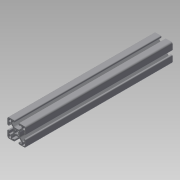
# Autodesk Inventor part: 1515-LS
Saved by Autodesk Inventor 2013 (Build 170138000, 138)
## iProperties
Created: 2014-04-23
Part Number: 1515-LS
Material: Generic
Document SubType Name: Modeling
Density: 1 g/cm^3
Vendor: 80/20 Inc.
Engineer: Ross Bowman
Designer: Ross Bowman
Catalog Web Link: 8020.net
Company: 80/20 Inc.
Author: Ross Bowman
Keywords: 80/20 , 8020 , T-Slot , Extrusion
Material: 6105-T5 Aluminum
Autodesk Inventor part; units mm, degrees
ref_plane "YZ Plane" through (0, 0, 0) normal (1, 0, 0) x (0, 1, 0)
ref_plane "XZ Plane" through (0, 0, 0) normal (0, 1, 0) x (-1, 0, 0)
ref_plane "XY Plane" through (0, 0, 0) normal (0, 0, 1) x (1, 0, 0)
sketch "Sketch1" plane through (0, 0, 0) normal (0, 0, 1) x (1, 0, 0)
  arc A0 (12.2428, 17.2466) -> (11.8618, 16.8656) centre (12.2428, 16.8656) ccw
  line L0 (14.4526, 17.2466) -> (12.2428, 17.2466)
  arc A1 (17.2466, 14.4526) -> (14.4526, 17.2466) centre (14.4526, 14.4526) ccw
  line L1 (17.2466, 12.2428) -> (17.2466, 14.4526)
  arc A2 (16.8656, 11.8618) -> (17.2466, 12.2428) centre (16.8656, 12.2428) ccw
  line L2 (12.2428, 11.8618) -> (16.8656, 11.8618)
  arc A3 (11.8618, 12.2428) -> (12.2428, 11.8618) centre (12.2428, 12.2428) ccw
  line L3 (11.8618, 16.8656) -> (11.8618, 12.2428)
  arc A4 (17.2466, -12.2428) -> (16.8656, -11.8618) centre (16.8656, -12.2428) ccw
  line L4 (17.2466, -14.4526) -> (17.2466, -12.2428)
  arc A5 (14.4526, -17.2466) -> (17.2466, -14.4526) centre (14.4526, -14.4526) ccw
  line L5 (12.2428, -17.2466) -> (14.4526, -17.2466)
  arc A6 (11.8618, -16.8656) -> (12.2428, -17.2466) centre (12.2428, -16.8656) ccw
  line L6 (11.8618, -12.2428) -> (11.8618, -16.8656)
  arc A7 (12.2428, -11.8618) -> (11.8618, -12.2428) centre (12.2428, -12.2428) ccw
  line L7 (16.8656, -11.8618) -> (12.2428, -11.8618)
  arc A8 (-12.2428, -17.2466) -> (-11.8618, -16.8656) centre (-12.2428, -16.8656) ccw
  line L8 (-14.4526, -17.2466) -> (-12.2428, -17.2466)
  arc A9 (-17.2466, -14.4526) -> (-14.4526, -17.2466) centre (-14.4526, -14.4526) ccw
  line L9 (-17.2466, -12.2428) -> (-17.2466, -14.4526)
  arc A10 (-16.8656, -11.8618) -> (-17.2466, -12.2428) centre (-16.8656, -12.2428) ccw
  line L10 (-12.2428, -11.8618) -> (-16.8656, -11.8618)
  arc A11 (-11.8618, -12.2428) -> (-12.2428, -11.8618) centre (-12.2428, -12.2428) ccw
  line L11 (-11.8618, -16.8656) -> (-11.8618, -12.2428)
  arc A12 (-17.2466, 12.2428) -> (-16.8656, 11.8618) centre (-16.8656, 12.2428) ccw
  line L12 (-17.2466, 14.4526) -> (-17.2466, 12.2428)
  arc A13 (-14.4526, 17.2466) -> (-17.2466, 14.4526) centre (-14.4526, 14.4526) ccw
  line L13 (-12.2428, 17.2466) -> (-14.4526, 17.2466)
  arc A14 (-11.8618, 16.8656) -> (-12.2428, 17.2466) centre (-12.2428, 16.8656) ccw
  line L14 (-11.8618, 12.2428) -> (-11.8618, 16.8656)
  arc A15 (-12.2428, 11.8618) -> (-11.8618, 12.2428) centre (-12.2428, 12.2428) ccw
  line L15 (-16.8656, 11.8618) -> (-12.2428, 11.8618)
  arc A16 (-4.3433, -2.7269) -> (-2.7269, -4.3433) centre (-3.5351, -3.5351) ccw
  line L16 (-2.9729, -1.3564) -> (-4.3433, -2.7269)
  arc A17 (-2.9729, 1.3564) -> (-2.9729, -1.3564) centre (0, 0) ccw
  line L17 (-4.3433, 2.7269) -> (-2.9729, 1.3564)
  arc A18 (-2.7269, 4.3433) -> (-4.3433, 2.7269) centre (-3.5351, 3.5351) ccw
  line L18 (-1.3564, 2.9729) -> (-2.7269, 4.3433)
  arc A19 (1.3564, 2.9729) -> (-1.3564, 2.9729) centre (0, 0) ccw
  line L19 (2.6398, 4.2456) -> (1.3564, 2.9729)
  arc A20 (4.2456, 2.6398) -> (2.6398, 4.2456) centre (3.5351, 3.5351) ccw
  line L20 (2.9729, 1.3564) -> (4.2456, 2.6398)
  arc A21 (2.9729, -1.3564) -> (2.9729, 1.3564) centre (0, 0) ccw
  line L21 (4.3433, -2.7269) -> (2.9729, -1.3564)
  arc A22 (2.7269, -4.3433) -> (4.3433, -2.7269) centre (3.5351, -3.5351) ccw
  line L22 (1.3564, -2.9729) -> (2.7269, -4.3433)
  arc A23 (-1.3564, -2.9729) -> (1.3564, -2.9729) centre (0, 0) ccw
  line L23 (-2.7269, -4.3433) -> (-1.3564, -2.9729)
  arc A24 (15.8242, -7.239) -> (15.4432, -6.858) centre (15.4432, -7.239) ccw
  line L24 (15.8242, -7.239) -> (15.8242, -9.013)
  arc A25 (14.5542, -10.287) -> (15.8242, -9.013) centre (14.5542, -9.017) ccw
  line L25 (14.5542, -10.287) -> (12.9683, -10.287)
  arc A26 (12.0703, -9.915) -> (12.9683, -10.287) centre (12.9683, -9.017) ccw
  line L26 (12.0703, -9.915) -> (8.1222, -5.9669)
  arc A27 (6.731, -2.6083) -> (8.1222, -5.9669) centre (11.4808, -2.6083) ccw
  line L27 (6.731, -2.6083) -> (6.731, 2.6083)
  arc A28 (8.1222, 5.9669) -> (6.731, 2.6083) centre (11.4808, 2.6083) ccw
  line L28 (8.1222, 5.9669) -> (12.0703, 9.915)
  arc A29 (12.9683, 10.287) -> (12.0703, 9.915) centre (12.9683, 9.017) ccw
  line L29 (12.9683, 10.287) -> (14.5542, 10.287)
  arc A30 (15.8242, 9.013) -> (14.5542, 10.287) centre (14.5542, 9.017) ccw
  line L30 (15.8242, 9.013) -> (15.8242, 7.239)
  arc A31 (15.4432, 6.858) -> (15.8242, 7.239) centre (15.4432, 7.239) ccw
  line L31 (15.4432, 6.858) -> (15.367, 6.858)
  arc A32 (15.367, 6.858) -> (14.986, 6.477) centre (15.367, 6.477) ccw
  line L32 (14.986, 6.477) -> (14.986, 5.6388)
  arc A33 (14.986, 5.6388) -> (16.5608, 4.064) centre (16.5608, 5.6388) ccw
  line L33 (16.5608, 4.064) -> (17.4752, 4.064)
  arc A34 (17.4752, 4.064) -> (19.05, 5.6388) centre (17.4752, 5.6388) ccw
  line L34 (19.05, 5.6388) -> (19.05, 15.875)
  arc A35 (19.05, 15.875) -> (15.875, 19.05) centre (15.875, 15.875) ccw
  line L35 (15.875, 19.05) -> (5.6388, 19.05)
  arc A36 (5.6388, 19.05) -> (4.064, 17.4752) centre (5.6388, 17.4752) ccw
  line L36 (4.064, 17.4752) -> (4.064, 16.5608)
  arc A37 (4.064, 16.5608) -> (5.6388, 14.986) centre (5.6388, 16.5608) ccw
  line L37 (5.6388, 14.986) -> (6.477, 14.986)
  arc A38 (6.477, 14.986) -> (6.858, 15.367) centre (6.477, 15.367) ccw
  line L38 (6.858, 15.367) -> (6.858, 15.4432)
  arc A39 (7.239, 15.8242) -> (6.858, 15.4432) centre (7.239, 15.4432) ccw
  line L39 (7.239, 15.8242) -> (9.013, 15.8242)
  arc A40 (10.287, 14.5542) -> (9.013, 15.8242) centre (9.017, 14.5542) ccw
  line L40 (10.287, 14.5542) -> (10.287, 12.9683)
  arc A41 (9.915, 12.0703) -> (10.287, 12.9683) centre (9.017, 12.9683) ccw
  line L41 (9.915, 12.0703) -> (5.9669, 8.1222)
  arc A42 (2.6083, 6.731) -> (5.9669, 8.1222) centre (2.6083, 11.4808) ccw
  line L42 (2.6083, 6.731) -> (-2.6083, 6.731)
  arc A43 (-5.9669, 8.1222) -> (-2.6083, 6.731) centre (-2.6083, 11.4808) ccw
  line L43 (-5.9669, 8.1222) -> (-9.915, 12.0703)
  arc A44 (-10.287, 12.9683) -> (-9.915, 12.0703) centre (-9.017, 12.9683) ccw
  line L44 (-10.287, 12.9683) -> (-10.287, 14.5542)
  arc A45 (-9.013, 15.8242) -> (-10.287, 14.5542) centre (-9.017, 14.5542) ccw
  line L45 (-9.013, 15.8242) -> (-7.239, 15.8242)
  arc A46 (-6.858, 15.4432) -> (-7.239, 15.8242) centre (-7.239, 15.4432) ccw
  line L46 (-6.858, 15.4432) -> (-6.858, 15.367)
  arc A47 (-6.858, 15.367) -> (-6.477, 14.986) centre (-6.477, 15.367) ccw
  line L47 (-6.477, 14.986) -> (-5.6388, 14.986)
  arc A48 (-5.6388, 14.986) -> (-4.064, 16.5608) centre (-5.6388, 16.5608) ccw
  line L48 (-4.064, 16.5608) -> (-4.064, 17.4752)
  arc A49 (-4.064, 17.4752) -> (-5.6388, 19.05) centre (-5.6388, 17.4752) ccw
  line L49 (-5.6388, 19.05) -> (-15.875, 19.05)
  arc A50 (-15.875, 19.05) -> (-19.05, 15.875) centre (-15.875, 15.875) ccw
  line L50 (-19.05, 15.875) -> (-19.05, 5.6388)
  arc A51 (-19.05, 5.6388) -> (-17.4752, 4.064) centre (-17.4752, 5.6388) ccw
  line L51 (-17.4752, 4.064) -> (-16.5608, 4.064)
  arc A52 (-16.5608, 4.064) -> (-14.986, 5.6388) centre (-16.5608, 5.6388) ccw
  line L52 (-14.986, 5.6388) -> (-14.986, 6.477)
  arc A53 (-14.986, 6.477) -> (-15.367, 6.858) centre (-15.367, 6.477) ccw
  line L53 (-15.367, 6.858) -> (-15.4432, 6.858)
  arc A54 (-15.8242, 7.239) -> (-15.4432, 6.858) centre (-15.4432, 7.239) ccw
  line L54 (-15.8242, 7.239) -> (-15.8242, 9.013)
  arc A55 (-14.5542, 10.287) -> (-15.8242, 9.013) centre (-14.5542, 9.017) ccw
  line L55 (-14.5542, 10.287) -> (-12.9683, 10.287)
  arc A56 (-12.0703, 9.915) -> (-12.9683, 10.287) centre (-12.9683, 9.017) ccw
  line L56 (-12.0703, 9.915) -> (-8.1222, 5.9669)
  arc A57 (-6.731, 2.6083) -> (-8.1222, 5.9669) centre (-11.4808, 2.6083) ccw
  line L57 (-6.731, 2.6083) -> (-6.731, -2.6083)
  arc A58 (-8.1222, -5.9669) -> (-6.731, -2.6083) centre (-11.4808, -2.6083) ccw
  line L58 (-8.1222, -5.9669) -> (-12.0703, -9.915)
  arc A59 (-12.9683, -10.287) -> (-12.0703, -9.915) centre (-12.9683, -9.017) ccw
  line L59 (-12.9683, -10.287) -> (-14.5542, -10.287)
  arc A60 (-15.8242, -9.013) -> (-14.5542, -10.287) centre (-14.5542, -9.017) ccw
  line L60 (-15.8242, -9.013) -> (-15.8242, -7.239)
  arc A61 (-15.4432, -6.858) -> (-15.8242, -7.239) centre (-15.4432, -7.239) ccw
  line L61 (-15.4432, -6.858) -> (-15.367, -6.858)
  arc A62 (-15.367, -6.858) -> (-14.986, -6.477) centre (-15.367, -6.477) ccw
  line L62 (-14.986, -6.477) -> (-14.986, -5.6388)
  arc A63 (-14.986, -5.6388) -> (-16.5608, -4.064) centre (-16.5608, -5.6388) ccw
  line L63 (-16.5608, -4.064) -> (-17.4752, -4.064)
  arc A64 (-17.4752, -4.064) -> (-19.05, -5.6388) centre (-17.4752, -5.6388) ccw
  line L64 (-19.05, -5.6388) -> (-19.05, -15.875)
  arc A65 (-19.05, -15.875) -> (-15.875, -19.05) centre (-15.875, -15.875) ccw
  line L65 (-15.875, -19.05) -> (-5.6388, -19.05)
  arc A66 (-5.6388, -19.05) -> (-4.064, -17.4752) centre (-5.6388, -17.4752) ccw
  line L66 (-4.064, -17.4752) -> (-4.064, -16.5608)
  arc A67 (-4.064, -16.5608) -> (-5.6388, -14.986) centre (-5.6388, -16.5608) ccw
  line L67 (-5.6388, -14.986) -> (-6.477, -14.986)
  arc A68 (-6.477, -14.986) -> (-6.858, -15.367) centre (-6.477, -15.367) ccw
  line L68 (-6.858, -15.367) -> (-6.858, -15.4432)
  arc A69 (-7.239, -15.8242) -> (-6.858, -15.4432) centre (-7.239, -15.4432) ccw
  line L69 (-7.239, -15.8242) -> (-9.013, -15.8242)
  arc A70 (-10.287, -14.5542) -> (-9.013, -15.8242) centre (-9.017, -14.5542) ccw
  line L70 (-10.287, -14.5542) -> (-10.287, -12.9683)
  arc A71 (-9.915, -12.0703) -> (-10.287, -12.9683) centre (-9.017, -12.9683) ccw
  line L71 (-9.915, -12.0703) -> (-5.9669, -8.1222)
  arc A72 (-2.6083, -6.731) -> (-5.9669, -8.1222) centre (-2.6083, -11.4808) ccw
  line L72 (-2.6083, -6.731) -> (2.6083, -6.731)
  arc A73 (5.9669, -8.1222) -> (2.6083, -6.731) centre (2.6083, -11.4808) ccw
  line L73 (5.9669, -8.1222) -> (9.915, -12.0703)
  arc A74 (10.287, -12.9683) -> (9.915, -12.0703) centre (9.017, -12.9683) ccw
  line L74 (10.287, -12.9683) -> (10.287, -14.5542)
  arc A75 (9.013, -15.8242) -> (10.287, -14.5542) centre (9.017, -14.5542) ccw
  line L75 (9.013, -15.8242) -> (7.239, -15.8242)
  arc A76 (6.858, -15.4432) -> (7.239, -15.8242) centre (7.239, -15.4432) ccw
  line L76 (6.858, -15.4432) -> (6.858, -15.367)
  arc A77 (6.858, -15.367) -> (6.477, -14.986) centre (6.477, -15.367) ccw
  line L77 (6.477, -14.986) -> (5.6388, -14.986)
  arc A78 (5.6388, -14.986) -> (4.064, -16.5608) centre (5.6388, -16.5608) ccw
  line L78 (4.064, -16.5608) -> (4.064, -17.4752)
  arc A79 (4.064, -17.4752) -> (5.6388, -19.05) centre (5.6388, -17.4752) ccw
  line L79 (5.6388, -19.05) -> (15.875, -19.05)
  arc A80 (15.875, -19.05) -> (19.05, -15.875) centre (15.875, -15.875) ccw
  line L80 (19.05, -15.875) -> (19.05, -5.6388)
  arc A81 (19.05, -5.6388) -> (17.4752, -4.064) centre (17.4752, -5.6388) ccw
  line L81 (17.4752, -4.064) -> (16.5608, -4.064)
  arc A82 (16.5608, -4.064) -> (14.986, -5.6388) centre (16.5608, -5.6388) ccw
  line L82 (14.986, -5.6388) -> (14.986, -6.477)
  arc A83 (14.986, -6.477) -> (15.367, -6.858) centre (15.367, -6.477) ccw
  line L83 (15.367, -6.858) -> (15.4432, -6.858)
  constraints: 168 end point, 168 point on circle, 84 centre point
extrude "Extrusion1" add sketch "Sketch1" against normal blind 304.8
body "Solid1"
